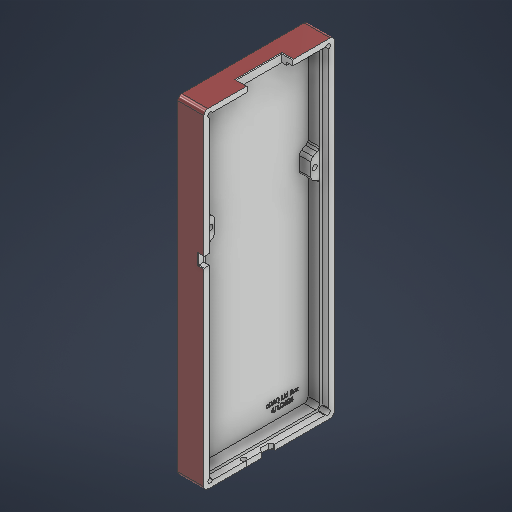
# Autodesk Inventor part: cDAQ_Lid_Box
Saved by Autodesk Inventor 2027 (Build 310192000, 192)
## iProperties
Created: 2026-05-08
Part Number: cDAQ_Lid_Box
Material: Generic
Document SubType Name: Modeling
Designer: giese
Density: 1 g/cm^3
Appearance: Default
Author: giese
Autodesk Inventor part; units mm, degrees
(part 1 of 2)
ref_plane "YZ Plane" through (0, 0, 0) normal (1, 0, 0) x (0, 1, 0)
ref_plane "XZ Plane" through (0, 0, 0) normal (0, 1, 0) x (-1, 0, 0)
ref_plane "XY Plane" through (0, 0, 0) normal (0, 0, 1) x (1, 0, 0)
sketch "Sketch1" plane through (0, 0, 0) normal (1, 0, 0) x (0, 1, 0)
  line L0 (50.7569, 48.4212) -> (-205.7831, 48.4212)
  line L1 (-205.7831, 48.4212) -> (-205.7831, -53.1788)
  line L2 (-205.7831, -53.1788) -> (50.7569, -53.1788)
  line L3 (50.7569, -53.1788) -> (50.7569, 48.4212)
  point P0 (0, 0)
  dimension "d0" = 101.6
  dimension "d1" = 256.54
  constraints: 8 end point, 2 parallel, 1 horizontal, 1 perpendicular
  measures "d0" distance of L2.end L0.start
  measures "d1" distance of L0.start L0.end
extrude "Extrusion1" add sketch "Sketch1" along normal blind 20.32
sketch "Sketch2" plane through (20.32, 0, 0) normal (1, 0, 0) x (0, 0, -1)
  line L0 (-42.0712, 44.4069) -> (46.8288, 44.4069)
  line L1 (46.8288, 44.4069) -> (46.8288, -199.4331)
  line L2 (46.8288, -199.4331) -> (-42.0712, -199.4331)
  line L3 (-42.0712, -199.4331) -> (-42.0712, 44.4069)
  line L4 (-48.4212, 50.7569) -> (-48.4212, -205.7831) projected
  line L5 (-48.4212, -205.7831) -> (53.1788, -205.7831) projected
  point P0 (0, 0)
  dimension "d4" = 88.9
  dimension "d5" = 243.84
  dimension "d6" = 6.35
  dimension "d7" = 6.35
  constraints: 8 end point, 2 parallel, 1 horizontal, 1 perpendicular
  measures "d4" distance of L0.start L0.end
  measures "d5" distance of L0.end L1.end
  measures "d6" distance between parallel lines of L4 L3
  measures "d7" distance between parallel lines of L5 L2
extrude "Extrusion2" cut sketch "Sketch2" against normal blind 13.97
sketch "Sketch3" plane through (0, 0, 0) normal (-1, 0, 0) x (0, 0, 1)
  circle A0 centre (-30.3188, 7.3229) radius 2
  line L0 (-53.1788, -205.7831) -> (-53.1788, 50.7569) projected
  line L1 (-53.1788, 50.7569) -> (48.4212, 50.7569) projected
  circle A1 centre (-11.82, 7.3229) radius 2
  circle A2 centre (6.6789, 7.3229) radius 2
  point P0 (0, 0)
  dimension "d10" = 22.86
  dimension "d11" = 43.434
  dimension "d12" = 43.434
  dimension "d13" = 18.4988
  dimension "d14" = 4
  dimension "d15" = 4
  dimension "d16" = 43.434
  dimension "d17" = 18.4988
  dimension "d18" = 36.9976
  dimension "d21" = 4
  constraints: 3 centre point
  measures "d10" distance from line of L0 A0.centre
  measures "d11" distance from line of L1 A0.centre
  measures "d12" distance from line of L1 A1.centre
  measures "d13" distance of A0.centre A1.centre
  measures "d14" diameter of A1
  measures "d15" diameter of A2
  measures "d16" distance from line of L1 A2.centre
  measures "d17" distance of A1.centre A2.centre
  measures "d18" distance of A0.centre A2.centre
  measures "d21" diameter of A0
extrude "Extrusion3" [suppressed]
sketch "Sketch6" plane through (0, 50.7569, 48.4212) normal (0, 1, 0) x (1, 0, 0)
  line L0 (20.32, 6.35) -> (20.32, 95.25) projected
  line L1 (11.684, 33.7719) -> (20.32, 33.7719)
  line L2 (20.32, 33.7719) -> (20.32, 69.342)
  line L3 (20.32, 69.342) -> (11.684, 69.342)
  line L4 (11.684, 69.342) -> (11.684, 33.7719)
  line L5 (0, 101.6) -> (20.32, 101.6) projected
  point P0 (0, 48.4212)
  point P1 (16.002, 69.342)
  point P2 (16.002, 33.7719)
  dimension "d30" = 8.636
  dimension "d31" = 35.5701
  dimension "d32" = 32.258
  constraints: 8 end point, 2 midpoint, 2 parallel, 1 horizontal, 1 perpendicular, 1 point on line
  measures "d30" distance between parallel lines of L0 L4
  measures "d31" distance of point (16.002, 69.342) point (16.002, 33.772)
  measures "d32" distance between parallel lines of L5 L3
extrude "Extrusion5" cut sketch "Sketch6" against normal blind 6.35
fillet "Fillet1" radius 3.175 4 edges at (10.16, 50.7569, -53.1788) (10.16, 50.7569, 48.4212) (10.16, -205.7831, 48.4212) (10.16, -205.7831, -53.1788)
sketch "Sketch7" plane through (20.32, 0, 0) normal (1, 0, 0) x (0, 0, -1)
  line L0 (-42.0712, -199.4331) -> (-42.0712, 44.4069) projected
  line L1 (-42.0712, 44.4069) -> (-42.3252, 44.4069)
  line L2 (-42.3252, 46.4643) -> (-44.1286, 46.4643)
  line L3 (-44.1286, 46.4643) -> (-44.1286, 51.0109)
  line L4 (-42.0712, -190.1621) -> (-42.0712, -199.4331)
  line L5 (46.8288, -199.4331) -> (-42.0712, -199.4331) projected
  line L6 (-40.4202, -201.4905) -> (-44.1286, -201.4905)
  line L7 (-44.1286, -201.4905) -> (-44.1286, -190.1621)
  line L8 (46.8288, 44.4069) -> (46.8288, -199.4331) projected
  line L9 (46.8288, -192.7021) -> (46.8288, -199.4331)
  line L10 (46.8288, -199.4331) -> (43.9078, -199.4331)
  line L11 (46.8288, -199.4331) -> (46.8288, -192.7021)
  line L12 (48.8862, -192.7021) -> (48.8862, -201.4905)
  line L13 (48.8862, -201.4905) -> (43.9078, -201.4905)
  line L14 (-42.0712, 44.4069) -> (46.8288, 44.4069) projected
  line L15 (42.0028, 44.4069) -> (46.8288, 44.4069)
  line L16 (48.8862, 48.4709) -> (48.8862, 46.4643)
  line L17 (48.8862, 46.4643) -> (42.0028, 46.4643)
  line L18 (-42.3252, 46.4643) -> (42.0028, 46.4643)
  line L19 (42.0028, 44.4069) -> (-42.3252, 44.4069)
  line L20 (48.8862, 48.4709) -> (48.8862, -192.7021)
  line L21 (44.2888, -195.2421) -> (44.2888, 44.4069)
  line L22 (43.9078, -199.4331) -> (-40.4202, -199.4331)
  line L23 (-40.4202, -201.4905) -> (43.9078, -201.4905)
  line L24 (-44.1286, -190.1621) -> (-44.1286, 51.0109)
  line L25 (-42.0712, 44.4069) -> (-42.0712, -190.1621)
  point P0 (0, 0)
  point P1 (-42.0712, 51.0109)
  point P2 (-44.2302, 48.9789)
  point P3 (46.8288, 48.4709)
  point P4 (48.8862, 46.4643)
  dimension "d34" = 2.0574
  dimension "d35" = 2.0574
  dimension "d38" = 2.0574
  dimension "d39" = 2.0574
  dimension "d42" = 2.0574
  dimension "d43" = 2.0574
  dimension "d46" = 2.0574
  dimension "d47" = 2.0574
  constraints: 44 end point, 9 point on line, 4 parallel, 4 perpendicular, 2 collinear, 2 horizontal, 2 vertical
  measures "d34" distance between parallel lines of L2 L1
  measures "d35" distance between parallel lines of L0 L3
  measures "d38" distance between parallel lines of L7 L0
  measures "d39" distance between parallel lines of L5 L6
  measures "d42" distance between parallel lines of L5 L13
  measures "d43" distance between parallel lines of L8 L12
  measures "d46" distance between parallel lines of L14 L17
  measures "d47" distance between parallel lines of L8 L16
extrude "Extrusion6" cut sketch "Sketch7" against normal blind 5 contours L0 L14 L8 L5 | L18 L17 L20 L12 L13 L23 L6 L7 L24 L2
fillet "Fillet2" radius 3.175 6 edges at (10.835, 44.4069, 42.0712) (10.835, 44.4069, -46.8288) (10.835, -199.4331, 42.0712) (17.82, -201.4905, 44.1286) (10.835, -199.4331, -46.8288) (17.82, -201.4905, -48.8862)
sketch "Sketch11" plane through (15.32, 0, 0) normal (1, 0, 0) x (0, 0, -1)
  circle A0 centre (48.0988, 45.6769) radius 1.9939
  line L0 (50.0038, 50.7569) -> (20.9208, 50.7569) projected
  line L1 (53.1788, -202.6081) -> (53.1788, 47.5819) projected
  arc A1 (46.9238, 45.7719) -> (43.7488, 48.9469) centre (43.7488, 45.7719) ccw projected
  circle A2 centre (-43.3412, 45.6769) radius 1.9939
  line L2 (-48.4212, 47.5819) -> (-48.4212, -202.6081) projected
  line L3 (-14.6493, 50.7569) -> (-45.2462, 50.7569) projected
  circle A3 centre (48.0988, -200.7031) radius 1.9939
  line L4 (-45.2462, -205.7831) -> (50.0038, -205.7831) projected
  circle A4 centre (-43.3412, -200.7031) radius 1.9939
  circle A5 centre (43.0188, -35.6031) radius 1.9939
  circle A6 centre (-38.2612, -35.6031) radius 1.9939
  point P0 (0, 0)
  point P1 (45.9939, 48.017)
  point P2 (48.5528, -43.2993)
  point P3 (45.3778, -46.4743)
  point P4 (-30.4007, -42.8803)
  point P5 (-33.5757, -46.0553)
  dimension "d58" = 3.9878
  dimension "d59" = 5.08
  dimension "d60" = 5.08
  dimension "d61" = 3.9878
  dimension "d62" = 3.9878
  dimension "d63" = 5.08
  dimension "d64" = 5.08
  dimension "d65" = 3.9878
  dimension "d66" = 5.08
  dimension "d67" = 5.08
  dimension "d76" = 5.08
  dimension "d77" = 5.08
  dimension "d114" = 3.9878
  dimension "d115" = 86.36
  dimension "d116" = 10.16
  dimension "d117" = 3.9878
  dimension "d118" = 86.36
  dimension "d119" = 10.16
  constraints: 6 centre point, 1 point on circle
  measures "d58" diameter of A0
  measures "d59" distance from line of L2 A2.centre
  measures "d60" distance from line of L3 A2.centre
  measures "d61" diameter of A2
  measures "d62" diameter of A3
  measures "d63" distance from line of L1 A3.centre
  measures "d64" distance from line of L4 A3.centre
  measures "d65" diameter of A4
  measures "d66" distance from line of L2 A4.centre
  measures "d67" distance from line of L4 A4.centre
  measures "d76" distance from line of L1 A0.centre
  measures "d77" distance from line of L0 A0.centre
  measures "d114" diameter of A5
  measures "d115" distance from line of A5.centre L0
  measures "d116" distance from line of L1 A5.centre
  measures "d117" diameter of A6
  measures "d118" distance from line of A6.centre L3
  measures "d119" distance from line of L2 A6.centre
extrude "Extrusion8" cut sketch "Sketch11" along normal blind 5.08 and the other way blind 17.78
sketch "Sketch13" plane through (6.35, 0, 0) normal (1, 0, 0) x (0, 0, -1)
  line L0 (14.1785, -185.2739) -> (39.2344, -185.2739) construction
  line L1 (39.2344, -185.2739) -> (39.2344, -194.1382) construction
  line L2 (39.2344, -194.1382) -> (14.1785, -194.1382) construction
  line L3 (14.1785, -194.1382) -> (14.1785, -185.2739) construction
  spline S0 degree 2 poles (15.3666, -188.5097) (15.1295, -188.5097) (14.7367, -188.3639) (14.5959, -188.2157) knots 0 0 0 1 2 2 2
  spline S1 degree 2 poles (14.5959, -188.2157) (14.4552, -188.07) (14.2995, -187.6205) (14.2995, -187.3191) knots 0 0 0 1 2 2 2
  spline S2 degree 2 poles (14.2995, -187.3191) (14.2995, -187.0178) (14.4601, -186.5781) (14.5959, -186.4299) knots 0 0 0 1 2 2 2
  spline S3 degree 2 poles (14.5959, -186.4299) (14.7318, -186.2792) (15.1344, -186.1187) (15.3666, -186.1187) knots 0 0 0 1 2 2 2
  spline S4 degree 2 poles (15.3666, -186.1187) (15.5543, -186.1187) (15.9051, -186.2249) (16.0409, -186.2941) knots 0 0 0 1 2 2 2
  line L4 (16.0409, -186.2941) -> (16.0409, -186.7263)
  line L5 (16.0409, -186.7263) -> (16.0187, -186.7263)
  spline S5 degree 2 poles (16.0187, -186.7263) (15.9767, -186.6917) (15.8482, -186.6028) (15.7569, -186.5559) knots 0 0 0 1 2 2 2
  spline S6 degree 2 poles (15.7569, -186.5559) (15.6753, -186.5164) (15.458, -186.4546) (15.3592, -186.4546) knots 0 0 0 1 2 2 2
  spline S7 degree 2 poles (15.3592, -186.4546) (15.0603, -186.4546) (14.6972, -186.9066) (14.6972, -187.3191) knots 0 0 0 1 2 2 2
  spline S8 degree 2 poles (14.6972, -187.3191) (14.6972, -187.7217) (15.048, -188.1737) (15.3592, -188.1737) knots 0 0 0 1 2 2 2
  spline S9 degree 2 poles (15.3592, -188.1737) (15.5469, -188.1737) (15.8878, -188.0181) (16.0187, -187.8971) knots 0 0 0 1 2 2 2
  line L6 (16.0187, -187.8971) -> (16.0409, -187.8971)
  line L7 (16.0409, -187.8971) -> (16.0409, -188.3293)
  spline S10 degree 2 poles (16.0409, -188.3293) (15.9841, -188.3565) (15.8112, -188.4331) (15.742, -188.4504) knots 0 0 0 1 2 2 2
  spline S11 degree 2 poles (15.742, -188.4504) (15.6432, -188.48) (15.4876, -188.5097) (15.3666, -188.5097) knots 0 0 0 1 2 2 2
  spline S12 degree 2 poles (18.8246, -186.9363) (18.8246, -187.3537) (18.4862, -188.0255) (18.2022, -188.2133) knots 0 0 0 1 2 2 2
  spline S13 degree 2 poles (18.2022, -188.2133) (17.97, -188.359) (17.4933, -188.4578) (17.1228, -188.4578) knots 0 0 0 1 2 2 2
  line L8 (17.1228, -188.4578) -> (16.4213, -188.4578)
  line L9 (16.4213, -188.4578) -> (16.4213, -185.4098)
  line L10 (16.4213, -185.4098) -> (17.1154, -185.4098)
  spline S14 degree 2 poles (17.1154, -185.4098) (17.5451, -185.4098) (18.0342, -185.5382) (18.2071, -185.6519) knots 0 0 0 1 2 2 2
  spline S15 degree 2 poles (18.2071, -185.6519) (18.501, -185.847) (18.8246, -186.4917) (18.8246, -186.9363) knots 0 0 0 1 2 2 2
  spline S16 degree 2 poles (18.4022, -186.9313) (18.4022, -186.5806) (18.1701, -186.0841) (17.9404, -185.9433) knots 0 0 0 1 2 2 2
  spline S17 degree 2 poles (17.9404, -185.9433) (17.7773, -185.847) (17.4093, -185.7605) (17.1351, -185.7605) knots 0 0 0 1 2 2 2
  line L11 (17.1351, -185.7605) -> (16.8264, -185.7605)
  line L12 (16.8264, -185.7605) -> (16.8264, -188.107)
  line L13 (16.8264, -188.107) -> (17.1351, -188.107)
  spline S18 degree 2 poles (17.1351, -188.107) (17.4044, -188.107) (17.8119, -188.0206) (17.9774, -187.9045) knots 0 0 0 1 2 2 2
  spline S19 degree 2 poles (17.9774, -187.9045) (18.1898, -187.7612) (18.4022, -187.287) (18.4022, -186.9313) knots 0 0 0 1 2 2 2
  line L14 (18.9358, -188.4578) -> (19.9633, -185.4098)
  line L15 (19.9633, -185.4098) -> (20.4622, -185.4098)
  line L16 (20.4622, -185.4098) -> (21.4898, -188.4578)
  line L17 (21.4898, -188.4578) -> (21.0625, -188.4578)
  line L18 (21.0625, -188.4578) -> (20.7858, -187.6056)
  line L19 (20.7858, -187.6056) -> (19.6224, -187.6056)
  line L20 (19.6224, -187.6056) -> (19.3458, -188.4578)
  line L21 (19.3458, -188.4578) -> (18.9358, -188.4578)
  line L22 (20.6747, -187.2598) -> (20.2029, -185.8248)
  line L23 (20.2029, -185.8248) -> (19.7336, -187.2598)
  line L24 (19.7336, -187.2598) -> (20.6747, -187.2598)
  spline S20 degree 2 poles (24.3105, -189.2037) (24.1994, -189.2309) (23.9573, -189.2605) (23.8363, -189.2605) knots 0 0 0 1 2 2 2
  spline S21 degree 2 poles (23.8363, -189.2605) (23.4929, -189.2605) (23.0656, -188.8777) (23.0459, -188.522) knots 0 0 0 1 2 2 2
  spline S22 degree 2 poles (23.0459, -188.522) (23.0187, -188.522) (22.9718, -188.522) (22.952, -188.522) knots 0 0 0 1 2 2 2
  spline S23 degree 2 poles (22.952, -188.522) (22.6433, -188.522) (22.1468, -188.3121) (21.9689, -188.107) knots 0 0 0 1 2 2 2
  spline S24 degree 2 poles (21.9689, -188.107) (21.7936, -187.9045) (21.6059, -187.3117) (21.6059, -186.9363) knots 0 0 0 1 2 2 2
  spline S25 degree 2 poles (21.6059, -186.9363) (21.6059, -186.5509) (21.796, -185.968) (21.9714, -185.7605) knots 0 0 0 1 2 2 2
  spline S26 degree 2 poles (21.9714, -185.7605) (22.1493, -185.5555) (22.6457, -185.3456) (22.952, -185.3456) knots 0 0 0 1 2 2 2
  spline S27 degree 2 poles (22.952, -185.3456) (23.2632, -185.3456) (23.7622, -185.5629) (23.9351, -185.7605) knots 0 0 0 1 2 2 2
  spline S28 degree 2 poles (23.9351, -185.7605) (24.108, -185.9606) (24.3006, -186.5559) (24.3006, -186.9363) knots 0 0 0 1 2 2 2
  spline S29 degree 2 poles (24.3006, -186.9363) (24.3006, -187.5291) (23.8387, -188.2997) (23.4361, -188.4356) knots 0 0 0 1 2 2 2
  spline S30 degree 2 poles (23.4361, -188.4356) (23.446, -188.5492) (23.5053, -188.732) (23.5522, -188.7838) knots 0 0 0 1 2 2 2
  spline S31 degree 2 poles (23.5522, -188.7838) (23.609, -188.8481) (23.7646, -188.9073) (23.903, -188.9073) knots 0 0 0 1 2 2 2
  spline S32 degree 2 poles (23.903, -188.9073) (23.9845, -188.9073) (24.2068, -188.8555) (24.2562, -188.8357) knots 0 0 0 1 2 2 2
  line L25 (24.2562, -188.8357) -> (24.3105, -188.8357)
  line L26 (24.3105, -188.8357) -> (24.3105, -189.2037)
  spline S33 degree 2 poles (23.8783, -186.9363) (23.8783, -186.6324) (23.7474, -186.1656) (23.6288, -186.0125) knots 0 0 0 1 2 2 2
  spline S34 degree 2 poles (23.6288, -186.0125) (23.5078, -185.8544) (23.1669, -185.6963) (22.9545, -185.6963) knots 0 0 0 1 2 2 2
  spline S35 degree 2 poles (22.9545, -185.6963) (22.7347, -185.6963) (22.4037, -185.8495) (22.2777, -186.0125) knots 0 0 0 1 2 2 2
  spline S36 degree 2 poles (22.2777, -186.0125) (22.1567, -186.1681) (22.0282, -186.6399) (22.0282, -186.9363) knots 0 0 0 1 2 2 2
  spline S37 degree 2 poles (22.0282, -186.9363) (22.0282, -187.5365) (22.5321, -188.1762) (22.9545, -188.1762) knots 0 0 0 1 2 2 2
  spline S38 degree 2 poles (22.9545, -188.1762) (23.3769, -188.1762) (23.8783, -187.5365) (23.8783, -186.9363) knots 0 0 0 1 2 2 2
  line L27 (27.8204, -188.4578) -> (26.0544, -188.4578)
  line L28 (26.0544, -188.4578) -> (26.0544, -185.4098)
  line L29 (26.0544, -185.4098) -> (26.4594, -185.4098)
  line L30 (26.4594, -185.4098) -> (26.4594, -188.0972)
  line L31 (26.4594, -188.0972) -> (27.8204, -188.0972)
  line L32 (27.8204, -188.0972) -> (27.8204, -188.4578)
  line L33 (28.5021, -188.4578) -> (28.1168, -188.4578)
  line L34 (28.1168, -188.4578) -> (28.1168, -186.1706)
  line L35 (28.1168, -186.1706) -> (28.5021, -186.1706)
  line L36 (28.5021, -186.1706) -> (28.5021, -188.4578)
  line L37 (28.5293, -185.7902) -> (28.0921, -185.7902)
  line L38 (28.0921, -185.7902) -> (28.0921, -185.39)
  line L39 (28.0921, -185.39) -> (28.5293, -185.39)
  line L40 (28.5293, -185.39) -> (28.5293, -185.7902)
  line L41 (30.8264, -188.4578) -> (30.4411, -188.4578)
  line L42 (30.4411, -188.4578) -> (30.4411, -188.2256)
  spline S39 degree 2 poles (30.4411, -188.2256) (30.3522, -188.2997) (30.2213, -188.3985) (30.1324, -188.4405) knots 0 0 0 1 2 2 2
  spline S40 degree 2 poles (30.1324, -188.4405) (30.0508, -188.48) (29.8755, -188.522) (29.7594, -188.522) knots 0 0 0 1 2 2 2
  spline S41 degree 2 poles (29.7594, -188.522) (29.5717, -188.522) (29.2555, -188.3664) (29.1443, -188.2157) knots 0 0 0 1 2 2 2
  spline S42 degree 2 poles (29.1443, -188.2157) (29.0332, -188.0651) (28.9097, -187.6205) (28.9097, -187.3315) knots 0 0 0 1 2 2 2
  spline S43 degree 2 poles (28.9097, -187.3315) (28.9097, -187.0301) (29.0653, -186.5905) (29.2012, -186.425) knots 0 0 0 1 2 2 2
  spline S44 degree 2 poles (29.2012, -186.425) (29.3271, -186.2768) (29.6803, -186.1063) (29.8755, -186.1063) knots 0 0 0 1 2 2 2
  spline S45 degree 2 poles (29.8755, -186.1063) (30.0459, -186.1063) (30.3003, -186.1829) (30.4411, -186.2619) knots 0 0 0 1 2 2 2
  line L43 (30.4411, -186.2619) -> (30.4411, -185.2739)
  line L44 (30.4411, -185.2739) -> (30.8264, -185.2739)
  line L45 (30.8264, -185.2739) -> (30.8264, -188.4578)
  line L46 (30.4411, -187.902) -> (30.4411, -186.5806)
  spline S46 degree 2 poles (30.4411, -186.5806) (30.2978, -186.5114) (30.0706, -186.4595) (29.9397, -186.4595) knots 0 0 0 1 2 2 2
  spline S47 degree 2 poles (29.9397, -186.4595) (29.6433, -186.4595) (29.3074, -186.9041) (29.3074, -187.3241) knots 0 0 0 1 2 2 2
  spline S48 degree 2 poles (29.3074, -187.3241) (29.3074, -187.7291) (29.5642, -188.1564) (29.8483, -188.1564) knots 0 0 0 1 2 2 2
  spline S49 degree 2 poles (29.8483, -188.1564) (29.999, -188.1564) (30.3053, -188.0181) (30.4411, -187.902) knots 0 0 0 1 2 2 2
  spline S50 degree 2 poles (34.7908, -187.5217) (34.7908, -187.7489) (34.6179, -188.0972) (34.4746, -188.2108) knots 0 0 0 1 2 2 2
  spline S51 degree 2 poles (34.4746, -188.2108) (34.3017, -188.3442) (33.909, -188.4578) (33.5978, -188.4578) knots 0 0 0 1 2 2 2
  line L47 (33.5978, -188.4578) -> (32.7234, -188.4578)
  line L48 (32.7234, -188.4578) -> (32.7234, -185.4098)
  line L49 (32.7234, -185.4098) -> (33.5311, -185.4098)
  spline S52 degree 2 poles (33.5311, -185.4098) (33.8571, -185.4098) (34.1832, -185.4518) (34.3314, -185.5333) knots 0 0 0 1 2 2 2
  spline S53 degree 2 poles (34.3314, -185.5333) (34.4969, -185.6197) (34.6475, -185.9038) (34.6475, -186.0965) knots 0 0 0 1 2 2 2
  spline S54 degree 2 poles (34.6475, -186.0965) (34.6475, -186.3113) (34.4203, -186.6522) (34.2202, -186.7485) knots 0 0 0 1 2 2 2
  line L50 (34.2202, -186.7485) -> (34.2202, -186.7634)
  spline S55 degree 2 poles (34.2202, -186.7634) (34.4919, -186.8375) (34.7908, -187.2302) (34.7908, -187.5217) knots 0 0 0 1 2 2 2
  spline S56 degree 2 poles (34.3684, -187.5389) (34.3684, -187.366) (34.2696, -187.1437) (34.1214, -187.0647) knots 0 0 0 1 2 2 2
  spline S57 degree 2 poles (34.1214, -187.0647) (34.0251, -187.0153) (33.7979, -186.9857) (33.5879, -186.9857) knots 0 0 0 1 2 2 2
  line L51 (33.5879, -186.9857) -> (33.1285, -186.9857)
  line L52 (33.1285, -186.9857) -> (33.1285, -188.112)
  line L53 (33.1285, -188.112) -> (33.457, -188.112)
  spline S58 degree 2 poles (33.457, -188.112) (33.7238, -188.112) (34.03, -188.0626) (34.1486, -187.9835) knots 0 0 0 1 2 2 2
  spline S59 degree 2 poles (34.1486, -187.9835) (34.2622, -187.902) (34.3684, -187.6995) (34.3684, -187.5389) knots 0 0 0 1 2 2 2
  spline S60 degree 2 poles (34.2252, -186.1533) (34.2252, -186.0446) (34.1511, -185.8816) (34.0696, -185.8346) knots 0 0 0 1 2 2 2
  spline S61 degree 2 poles (34.0696, -185.8346) (33.9708, -185.7803) (33.7312, -185.7556) (33.5163, -185.7556) knots 0 0 0 1 2 2 2
  line L54 (33.5163, -185.7556) -> (33.1285, -185.7556)
  line L55 (33.1285, -185.7556) -> (33.1285, -186.6473)
  line L56 (33.1285, -186.6473) -> (33.5879, -186.6473)
  spline S62 degree 2 poles (33.5879, -186.6473) (33.7781, -186.6473) (33.9584, -186.6077) (34.0547, -186.546) knots 0 0 0 1 2 2 2
  spline S63 degree 2 poles (34.0547, -186.546) (34.1486, -186.4867) (34.2252, -186.2965) (34.2252, -186.1533) knots 0 0 0 1 2 2 2
  spline S64 degree 2 poles (37.0435, -187.3142) (37.0435, -187.8922) (36.4877, -188.522) (36.0233, -188.522) knots 0 0 0 1 2 2 2
  spline S65 degree 2 poles (36.0233, -188.522) (35.5466, -188.522) (35.0008, -187.8724) (35.0008, -187.3142) knots 0 0 0 1 2 2 2
  spline S66 degree 2 poles (35.0008, -187.3142) (35.0008, -186.7411) (35.5639, -186.1063) (36.0233, -186.1063) knots 0 0 0 1 2 2 2
  spline S67 degree 2 poles (36.0233, -186.1063) (36.4877, -186.1063) (37.0435, -186.7387) (37.0435, -187.3142) knots 0 0 0 1 2 2 2
  spline S68 degree 2 poles (36.6458, -187.3142) (36.6458, -186.8696) (36.3222, -186.4373) (36.0233, -186.4373) knots 0 0 0 1 2 2 2
  spline S69 degree 2 poles (36.0233, -186.4373) (35.7245, -186.4373) (35.3984, -186.8696) (35.3984, -187.3142) knots 0 0 0 1 2 2 2
  spline S70 degree 2 poles (35.3984, -187.3142) (35.3984, -187.7464) (35.7245, -188.191) (36.0233, -188.191) knots 0 0 0 1 2 2 2
  spline S71 degree 2 poles (36.0233, -188.191) (36.3197, -188.191) (36.6458, -187.7538) (36.6458, -187.3142) knots 0 0 0 1 2 2 2
  line L57 (39.2146, -188.4578) -> (38.7428, -188.4578)
  line L58 (38.7428, -188.4578) -> (38.1871, -187.5982)
  line L59 (38.1871, -187.5982) -> (37.6165, -188.4578)
  line L60 (37.6165, -188.4578) -> (37.1793, -188.4578)
  line L61 (37.1793, -188.4578) -> (37.9722, -187.3241)
  line L62 (37.9722, -187.3241) -> (37.1867, -186.1706)
  line L63 (37.1867, -186.1706) -> (37.6585, -186.1706)
  line L64 (37.6585, -186.1706) -> (38.2118, -187.0227)
  line L65 (38.2118, -187.0227) -> (38.7774, -186.1706)
  line L66 (38.7774, -186.1706) -> (39.2146, -186.1706)
  line L67 (39.2146, -186.1706) -> (38.4267, -187.2994)
  line L68 (38.4267, -187.2994) -> (39.2146, -188.4578)
  spline S72 degree 2 poles (20.3906, -192.4882) (20.3906, -192.7229) (20.235, -193.1206) (20.1041, -193.2539) knots 0 0 0 1 2 2 2
  spline S73 degree 2 poles (20.1041, -193.2539) (19.9682, -193.3947) (19.6274, -193.5405) (19.4224, -193.5405) knots 0 0 0 1 2 2 2
  spline S74 degree 2 poles (19.4224, -193.5405) (19.2173, -193.5405) (18.879, -193.4021) (18.7505, -193.2638) knots 0 0 0 1 2 2 2
  spline S75 degree 2 poles (18.7505, -193.2638) (18.5924, -193.0983) (18.4146, -192.5426) (18.4146, -192.1375) knots 0 0 0 1 2 2 2
  spline S76 degree 2 poles (18.4146, -192.1375) (18.4146, -191.7398) (18.5776, -191.1001) (18.748, -190.863) knots 0 0 0 1 2 2 2
  spline S77 degree 2 poles (18.748, -190.863) (18.9135, -190.6308) (19.4372, -190.3714) (19.7805, -190.3714) knots 0 0 0 1 2 2 2
  spline S78 degree 2 poles (19.7805, -190.3714) (19.8818, -190.3714) (20.0596, -190.3912) (20.1263, -190.4134) knots 0 0 0 1 2 2 2
  line L69 (20.1263, -190.4134) -> (20.1263, -190.8062)
  line L70 (20.1263, -190.8062) -> (20.109, -190.8062)
  spline S79 degree 2 poles (20.109, -190.8062) (20.0522, -190.7765) (19.8447, -190.7246) (19.7262, -190.7246) knots 0 0 0 1 2 2 2
  spline S80 degree 2 poles (19.7262, -190.7246) (19.3458, -190.7246) (18.879, -191.2384) (18.8345, -191.7423) knots 0 0 0 1 2 2 2
  spline S81 degree 2 poles (18.8345, -191.7423) (18.9802, -191.641) (19.2865, -191.5299) (19.4693, -191.5299) knots 0 0 0 1 2 2 2
  spline S82 degree 2 poles (19.4693, -191.5299) (19.6471, -191.5299) (19.9139, -191.6015) (20.0596, -191.7102) knots 0 0 0 1 2 2 2
  spline S83 degree 2 poles (20.0596, -191.7102) (20.2276, -191.8362) (20.3906, -192.2264) (20.3906, -192.4882) knots 0 0 0 1 2 2 2
  spline S84 degree 2 poles (19.9756, -192.5055) (19.9756, -192.3178) (19.8768, -192.0634) (19.7682, -191.9745) knots 0 0 0 1 2 2 2
  spline S85 degree 2 poles (19.7682, -191.9745) (19.6867, -191.9103) (19.4841, -191.8683) (19.3779, -191.8683) knots 0 0 0 1 2 2 2
  spline S86 degree 2 poles (19.3779, -191.8683) (19.2346, -191.8683) (18.9654, -191.9547) (18.8345, -192.0362) knots 0 0 0 1 2 2 2
  spline S87 degree 2 poles (18.8345, -192.0362) (18.832, -192.0807) (18.8271, -192.1647) (18.8271, -192.2289) knots 0 0 0 1 2 2 2
  spline S88 degree 2 poles (18.8271, -192.2289) (18.8271, -192.545) (18.9506, -192.9328) (19.0444, -193.0341) knots 0 0 0 1 2 2 2
  spline S89 degree 2 poles (19.0444, -193.0341) (19.1309, -193.1304) (19.3186, -193.207) (19.4248, -193.207) knots 0 0 0 1 2 2 2
  spline S90 degree 2 poles (19.4248, -193.207) (19.6718, -193.207) (19.9756, -192.8563) (19.9756, -192.5055) knots 0 0 0 1 2 2 2
  line L71 (22.0183, -190.2924) -> (20.8253, -194.1382)
  line L72 (20.8253, -194.1382) -> (20.4795, -194.1382)
  line L73 (20.4795, -194.1382) -> (21.6676, -190.2924)
  line L74 (21.6676, -190.2924) -> (22.0183, -190.2924)
  line L75 (24.0808, -193.4762) -> (22.5939, -193.4762)
  line L76 (22.5939, -193.4762) -> (22.5939, -193.165)
  line L77 (22.5939, -193.165) -> (23.1471, -193.165)
  line L78 (23.1471, -193.165) -> (23.1471, -191.1223)
  line L79 (23.1471, -191.1223) -> (22.5939, -191.1223)
  line L80 (22.5939, -191.1223) -> (22.5939, -190.8432)
  spline S91 degree 2 poles (22.5939, -190.8432) (22.9076, -190.8432) (23.204, -190.6654) (23.2237, -190.4184) knots 0 0 0 1 2 2 2
  line L81 (23.2237, -190.4184) -> (23.5399, -190.4184)
  line L82 (23.5399, -190.4184) -> (23.5399, -193.165)
  line L83 (23.5399, -193.165) -> (24.0808, -193.165)
  line L84 (24.0808, -193.165) -> (24.0808, -193.4762)
  line L85 (25.9086, -190.2924) -> (24.7156, -194.1382)
  line L86 (24.7156, -194.1382) -> (24.3698, -194.1382)
  line L87 (24.3698, -194.1382) -> (25.5579, -190.2924)
  line L88 (25.5579, -190.2924) -> (25.9086, -190.2924)
  line L89 (28.1242, -193.4762) -> (26.2445, -193.4762)
  line L90 (26.2445, -193.4762) -> (26.2445, -193.044)
  spline S92 degree 2 poles (26.2445, -193.044) (26.4471, -192.8538) (26.8077, -192.5006) (26.9806, -192.3104) knots 0 0 0 1 2 2 2
  spline S93 degree 2 poles (26.9806, -192.3104) (27.3289, -191.9275) (27.5833, -191.4681) (27.5833, -191.2236) knots 0 0 0 1 2 2 2
  spline S94 degree 2 poles (27.5833, -191.2236) (27.5833, -191.0951) (27.5043, -190.9025) (27.4326, -190.8407) knots 0 0 0 1 2 2 2
  spline S95 degree 2 poles (27.4326, -190.8407) (27.361, -190.779) (27.1733, -190.7172) (27.0597, -190.7172) knots 0 0 0 1 2 2 2
  spline S96 degree 2 poles (27.0597, -190.7172) (26.951, -190.7172) (26.7287, -190.7716) (26.6274, -190.8136) knots 0 0 0 1 2 2 2
  spline S97 degree 2 poles (26.6274, -190.8136) (26.5409, -190.8481) (26.3804, -190.9469) (26.331, -190.9815) knots 0 0 0 1 2 2 2
  line L91 (26.331, -190.9815) -> (26.3088, -190.9815)
  line L92 (26.3088, -190.9815) -> (26.3088, -190.5468)
  spline S98 degree 2 poles (26.3088, -190.5468) (26.4347, -190.4851) (26.8867, -190.364) (27.0893, -190.364) knots 0 0 0 1 2 2 2
  spline S99 degree 2 poles (27.0893, -190.364) (27.5166, -190.364) (27.9983, -190.816) (27.9983, -191.2014) knots 0 0 0 1 2 2 2
  spline S100 degree 2 poles (27.9983, -191.2014) (27.9983, -191.3817) (27.9143, -191.683) (27.8402, -191.8114) knots 0 0 0 1 2 2 2
  spline S101 degree 2 poles (27.8402, -191.8114) (27.7661, -191.9448) (27.5512, -192.2067) (27.4326, -192.3326) knots 0 0 0 1 2 2 2
  spline S102 degree 2 poles (27.4326, -192.3326) (27.24, -192.5426) (26.7682, -192.9921) (26.6274, -193.123) knots 0 0 0 1 2 2 2
  line L93 (26.6274, -193.123) -> (28.1242, -193.123)
  line L94 (28.1242, -193.123) -> (28.1242, -193.4762)
  spline S103 degree 2 poles (30.4288, -191.9522) (30.4288, -192.7723) (29.952, -193.5405) (29.4556, -193.5405) knots 0 0 0 1 2 2 2
  spline S104 degree 2 poles (29.4556, -193.5405) (28.9517, -193.5405) (28.4799, -192.7575) (28.4799, -191.9547) knots 0 0 0 1 2 2 2
  spline S105 degree 2 poles (28.4799, -191.9547) (28.4799, -191.1297) (28.9566, -190.3665) (29.4556, -190.3665) knots 0 0 0 1 2 2 2
  spline S106 degree 2 poles (29.4556, -190.3665) (29.957, -190.3665) (30.4288, -191.1569) (30.4288, -191.9522) knots 0 0 0 1 2 2 2
  spline S107 degree 2 poles (29.9051, -192.881) (29.9644, -192.7303) (30.0138, -192.2659) (30.0138, -191.9522) knots 0 0 0 1 2 2 2
  spline S108 degree 2 poles (30.0138, -191.9522) (30.0138, -191.6385) (29.9644, -191.1767) (29.9026, -191.021) knots 0 0 0 1 2 2 2
  spline S109 degree 2 poles (29.9026, -191.021) (29.8409, -190.8654) (29.626, -190.7049) (29.4556, -190.7049) knots 0 0 0 1 2 2 2
  spline S110 degree 2 poles (29.4556, -190.7049) (29.2851, -190.7049) (29.0653, -190.8654) (29.0011, -191.026) knots 0 0 0 1 2 2 2
  spline S111 degree 2 poles (29.0011, -191.026) (28.9393, -191.1816) (28.8949, -191.6558) (28.8949, -191.9547) knots 0 0 0 1 2 2 2
  spline S112 degree 2 poles (28.8949, -191.9547) (28.8949, -192.2758) (28.9344, -192.7056) (28.9986, -192.8736) knots 0 0 0 1 2 2 2
  spline S113 degree 2 poles (28.9986, -192.8736) (29.0579, -193.0316) (29.2777, -193.2021) (29.4556, -193.2021) knots 0 0 0 1 2 2 2
  spline S114 degree 2 poles (29.4556, -193.2021) (29.6235, -193.2021) (29.8434, -193.0415) (29.9051, -192.881) knots 0 0 0 1 2 2 2
  line L95 (32.6987, -193.4762) -> (30.819, -193.4762)
  line L96 (30.819, -193.4762) -> (30.819, -193.044)
  spline S115 degree 2 poles (30.819, -193.044) (31.0216, -192.8538) (31.3822, -192.5006) (31.5551, -192.3104) knots 0 0 0 1 2 2 2
  spline S116 degree 2 poles (31.5551, -192.3104) (31.9034, -191.9275) (32.1578, -191.4681) (32.1578, -191.2236) knots 0 0 0 1 2 2 2
  spline S117 degree 2 poles (32.1578, -191.2236) (32.1578, -191.0951) (32.0787, -190.9025) (32.0071, -190.8407) knots 0 0 0 1 2 2 2
  spline S118 degree 2 poles (32.0071, -190.8407) (31.9355, -190.779) (31.7477, -190.7172) (31.6341, -190.7172) knots 0 0 0 1 2 2 2
  spline S119 degree 2 poles (31.6341, -190.7172) (31.5254, -190.7172) (31.3031, -190.7716) (31.2019, -190.8136) knots 0 0 0 1 2 2 2
  spline S120 degree 2 poles (31.2019, -190.8136) (31.1154, -190.8481) (30.9549, -190.9469) (30.9055, -190.9815) knots 0 0 0 1 2 2 2
  line L97 (30.9055, -190.9815) -> (30.8832, -190.9815)
  line L98 (30.8832, -190.9815) -> (30.8832, -190.5468)
  spline S121 degree 2 poles (30.8832, -190.5468) (31.0092, -190.4851) (31.4612, -190.364) (31.6638, -190.364) knots 0 0 0 1 2 2 2
  spline S122 degree 2 poles (31.6638, -190.364) (32.0911, -190.364) (32.5727, -190.816) (32.5727, -191.2014) knots 0 0 0 1 2 2 2
  spline S123 degree 2 poles (32.5727, -191.2014) (32.5727, -191.3817) (32.4887, -191.683) (32.4146, -191.8114) knots 0 0 0 1 2 2 2
  spline S124 degree 2 poles (32.4146, -191.8114) (32.3405, -191.9448) (32.1257, -192.2067) (32.0071, -192.3326) knots 0 0 0 1 2 2 2
  spline S125 degree 2 poles (32.0071, -192.3326) (31.8144, -192.5426) (31.3427, -192.9921) (31.2019, -193.123) knots 0 0 0 1 2 2 2
  line L99 (31.2019, -193.123) -> (32.6987, -193.123)
  line L100 (32.6987, -193.123) -> (32.6987, -193.4762)
  spline S126 degree 2 poles (35.0329, -192.4882) (35.0329, -192.7229) (34.8773, -193.1206) (34.7463, -193.2539) knots 0 0 0 1 2 2 2
  spline S127 degree 2 poles (34.7463, -193.2539) (34.6105, -193.3947) (34.2696, -193.5405) (34.0646, -193.5405) knots 0 0 0 1 2 2 2
  spline S128 degree 2 poles (34.0646, -193.5405) (33.8596, -193.5405) (33.5212, -193.4021) (33.3928, -193.2638) knots 0 0 0 1 2 2 2
  spline S129 degree 2 poles (33.3928, -193.2638) (33.2347, -193.0983) (33.0569, -192.5426) (33.0569, -192.1375) knots 0 0 0 1 2 2 2
  spline S130 degree 2 poles (33.0569, -192.1375) (33.0569, -191.7398) (33.2199, -191.1001) (33.3903, -190.863) knots 0 0 0 1 2 2 2
  spline S131 degree 2 poles (33.3903, -190.863) (33.5558, -190.6308) (34.0794, -190.3714) (34.4228, -190.3714) knots 0 0 0 1 2 2 2
  spline S132 degree 2 poles (34.4228, -190.3714) (34.524, -190.3714) (34.7019, -190.3912) (34.7686, -190.4134) knots 0 0 0 1 2 2 2
  line L101 (34.7686, -190.4134) -> (34.7686, -190.8062)
  line L102 (34.7686, -190.8062) -> (34.7513, -190.8062)
  spline S133 degree 2 poles (34.7513, -190.8062) (34.6945, -190.7765) (34.487, -190.7246) (34.3684, -190.7246) knots 0 0 0 1 2 2 2
  spline S134 degree 2 poles (34.3684, -190.7246) (33.988, -190.7246) (33.5212, -191.2384) (33.4768, -191.7423) knots 0 0 0 1 2 2 2
  spline S135 degree 2 poles (33.4768, -191.7423) (33.6225, -191.641) (33.9288, -191.5299) (34.1115, -191.5299) knots 0 0 0 1 2 2 2
  spline S136 degree 2 poles (34.1115, -191.5299) (34.2894, -191.5299) (34.5562, -191.6015) (34.7019, -191.7102) knots 0 0 0 1 2 2 2
  spline S137 degree 2 poles (34.7019, -191.7102) (34.8698, -191.8362) (35.0329, -192.2264) (35.0329, -192.4882) knots 0 0 0 1 2 2 2
  spline S138 degree 2 poles (34.6179, -192.5055) (34.6179, -192.3178) (34.5191, -192.0634) (34.4104, -191.9745) knots 0 0 0 1 2 2 2
  spline S139 degree 2 poles (34.4104, -191.9745) (34.3289, -191.9103) (34.1264, -191.8683) (34.0202, -191.8683) knots 0 0 0 1 2 2 2
  spline S140 degree 2 poles (34.0202, -191.8683) (33.8769, -191.8683) (33.6077, -191.9547) (33.4768, -192.0362) knots 0 0 0 1 2 2 2
  spline S141 degree 2 poles (33.4768, -192.0362) (33.4743, -192.0807) (33.4693, -192.1647) (33.4693, -192.2289) knots 0 0 0 1 2 2 2
  spline S142 degree 2 poles (33.4693, -192.2289) (33.4693, -192.545) (33.5928, -192.9328) (33.6867, -193.0341) knots 0 0 0 1 2 2 2
  spline S143 degree 2 poles (33.6867, -193.0341) (33.7732, -193.1304) (33.9609, -193.207) (34.0671, -193.207) knots 0 0 0 1 2 2 2
  spline S144 degree 2 poles (34.0671, -193.207) (34.3141, -193.207) (34.6179, -192.8563) (34.6179, -192.5055) knots 0 0 0 1 2 2 2
  point P0 (0, 0)
  constraints: 2 other
emboss "Emboss1" sketch "Sketch13" operation cut depth 2.54 direction (-1, 0, 0)
sketch "Sketch14" plane through (0, 0, 0) normal (-1, 0, 0) x (0, 0, 1)
  line L0 (-10.4499, -187.9273) -> (8.7669, -187.9273) construction
  line L1 (8.7669, -187.9273) -> (8.7669, -196.7101) construction
  line L2 (8.7669, -196.7101) -> (-10.4499, -196.7101) construction
  line L3 (-10.4499, -196.7101) -> (-10.4499, -187.9273) construction
  line L4 (-23.4175, -195.887) -> (-20.8486, -188.267)
  line L5 (-20.8486, -188.267) -> (-19.6013, -188.267)
  line L6 (-19.6013, -188.267) -> (-17.0325, -195.887)
  line L7 (-17.0325, -195.887) -> (-18.1008, -195.887)
  line L8 (-18.1008, -195.887) -> (-18.7924, -193.7566)
  line L9 (-18.7924, -193.7566) -> (-21.7008, -193.7566)
  line L10 (-21.7008, -193.7566) -> (-22.3924, -195.887)
  line L11 (-22.3924, -195.887) -> (-23.4175, -195.887)
  line L12 (-19.0702, -192.8921) -> (-20.2497, -189.3044)
  line L13 (-20.2497, -189.3044) -> (-21.4229, -192.8921)
  line L14 (-21.4229, -192.8921) -> (-19.0702, -192.8921)
  line L15 (-10.4128, -195.887) -> (-11.7281, -195.887)
  line L16 (-11.7281, -195.887) -> (-14.1364, -192.855)
  line L17 (-14.1364, -192.855) -> (-15.2973, -192.855)
  line L18 (-15.2973, -192.855) -> (-15.2973, -195.887)
  line L19 (-15.2973, -195.887) -> (-16.31, -195.887)
  line L20 (-16.31, -195.887) -> (-16.31, -188.267)
  line L21 (-16.31, -188.267) -> (-14.3463, -188.267)
  spline S0 degree 2 poles (-14.3463, -188.267) (-13.6918, -188.267) (-12.8087, -188.409) (-12.4074, -188.6683) knots 0 0 0 1 2 2 2
  spline S1 degree 2 poles (-12.4074, -188.6683) (-12.006, -188.9277) (-11.5429, -189.7366) (-11.5429, -190.3356) knots 0 0 0 1 2 2 2
  spline S2 degree 2 poles (-11.5429, -190.3356) (-11.5429, -191.1692) (-12.395, -192.2993) (-13.1237, -192.571) knots 0 0 0 1 2 2 2
  line L22 (-13.1237, -192.571) -> (-10.4128, -195.887)
  spline S3 degree 2 poles (-12.5988, -190.4159) (-12.5988, -190.0824) (-12.8334, -189.5699) (-13.0804, -189.4032) knots 0 0 0 1 2 2 2
  spline S4 degree 2 poles (-13.0804, -189.4032) (-13.2966, -189.2612) (-13.8708, -189.1438) (-14.2907, -189.1438) knots 0 0 0 1 2 2 2
  line L23 (-14.2907, -189.1438) -> (-15.2973, -189.1438)
  line L24 (-15.2973, -189.1438) -> (-15.2973, -192.009)
  line L25 (-15.2973, -192.009) -> (-14.4081, -192.009)
  spline S5 degree 2 poles (-14.4081, -192.009) (-13.9696, -192.009) (-13.2719, -191.8547) (-13.031, -191.6138) knots 0 0 0 1 2 2 2
  spline S6 degree 2 poles (-13.031, -191.6138) (-12.8087, -191.4039) (-12.5988, -190.8111) (-12.5988, -190.4159) knots 0 0 0 1 2 2 2
  line L26 (-8.0293, -195.887) -> (-8.0293, -189.1685)
  line L27 (-8.0293, -189.1685) -> (-10.5857, -189.1685)
  line L28 (-10.5857, -189.1685) -> (-10.5857, -188.267)
  line L29 (-10.5857, -188.267) -> (-4.4601, -188.267)
  line L30 (-4.4601, -188.267) -> (-4.4601, -189.1685)
  line L31 (-4.4601, -189.1685) -> (-7.0166, -189.1685)
  line L32 (-7.0166, -189.1685) -> (-7.0166, -195.887)
  line L33 (-7.0166, -195.887) -> (-8.0293, -195.887)
  spline S7 degree 2 poles (-1.564, -196.0228) (-2.3914, -196.0228) (-3.5524, -195.677) (-4.0649, -195.43) knots 0 0 0 1 2 2 2
  line L34 (-4.0649, -195.43) -> (-4.0649, -194.158)
  line L35 (-4.0649, -194.158) -> (-3.9908, -194.158)
  spline S8 degree 2 poles (-3.9908, -194.158) (-3.4906, -194.6273) (-2.2247, -195.146) (-1.6381, -195.146) knots 0 0 0 1 2 2 2
  spline S9 degree 2 poles (-1.6381, -195.146) (-0.7983, -195.146) (0.06, -194.4482) (0.06, -193.8739) knots 0 0 0 1 2 2 2
  spline S10 degree 2 poles (0.06, -193.8739) (0.06, -193.417) (-0.3907, -192.8489) (-0.8786, -192.7068) knots 0 0 0 1 2 2 2
  spline S11 degree 2 poles (-0.8786, -192.7068) (-1.2305, -192.608) (-1.8172, -192.4722) (-2.2556, -192.361) knots 0 0 0 1 2 2 2
  spline S12 degree 2 poles (-2.2556, -192.361) (-2.6508, -192.256) (-3.2745, -191.9411) (-3.5153, -191.6879) knots 0 0 0 1 2 2 2
  spline S13 degree 2 poles (-3.5153, -191.6879) (-3.75, -191.4348) (-4.0093, -190.7555) (-4.0093, -190.3109) knots 0 0 0 1 2 2 2
  spline S14 degree 2 poles (-4.0093, -190.3109) (-4.0093, -189.3847) (-2.5643, -188.1311) (-1.4467, -188.1311) knots 0 0 0 1 2 2 2
  spline S15 degree 2 poles (-1.4467, -188.1311) (-0.8045, -188.1311) (0.3317, -188.3843) (0.8196, -188.6251) knots 0 0 0 1 2 2 2
  line L36 (0.8196, -188.6251) -> (0.8196, -189.8354)
  line L37 (0.8196, -189.8354) -> (0.7455, -189.8354)
  spline S16 degree 2 poles (0.7455, -189.8354) (0.3811, -189.502) (-0.7551, -189.008) (-1.3787, -189.008) knots 0 0 0 1 2 2 2
  spline S17 degree 2 poles (-1.3787, -189.008) (-2.0827, -189.008) (-2.9534, -189.6687) (-2.9534, -190.2059) knots 0 0 0 1 2 2 2
  spline S18 degree 2 poles (-2.9534, -190.2059) (-2.9534, -190.6876) (-2.4408, -191.2619) (-1.9592, -191.3915) knots 0 0 0 1 2 2 2
  spline S19 degree 2 poles (-1.9592, -191.3915) (-1.6381, -191.478) (-0.7057, -191.7003) (-0.3969, -191.7929) knots 0 0 0 1 2 2 2
  spline S20 degree 2 poles (-0.3969, -191.7929) (0.3873, -192.0337) (1.116, -193.0032) (1.116, -193.7134) knots 0 0 0 1 2 2 2
  spline S21 degree 2 poles (1.116, -193.7134) (1.116, -194.1641) (0.7516, -195.0286) (0.4244, -195.3312) knots 0 0 0 1 2 2 2
  spline S22 degree 2 poles (0.4244, -195.3312) (0.06, -195.6647) (-0.8662, -196.0228) (-1.564, -196.0228) knots 0 0 0 1 2 2 2
  line L38 (4.7222, -193.0156) -> (1.8385, -193.0156)
  line L39 (1.8385, -193.0156) -> (1.8385, -192.0893)
  line L40 (1.8385, -192.0893) -> (4.7222, -192.0893)
  line L41 (4.7222, -192.0893) -> (4.7222, -193.0156)
  line L42 (10.3662, -195.887) -> (5.951, -195.887)
  line L43 (5.951, -195.887) -> (5.951, -188.267)
  line L44 (5.951, -188.267) -> (6.9637, -188.267)
  line L45 (6.9637, -188.267) -> (6.9637, -194.9854)
  line L46 (6.9637, -194.9854) -> (10.3662, -194.9854)
  line L47 (10.3662, -194.9854) -> (10.3662, -195.887)
  spline S23 degree 2 poles (14.275, -195.2818) (14.1577, -195.3683) (13.7625, -195.677) (13.5772, -195.7696) knots 0 0 0 1 2 2 2
  spline S24 degree 2 poles (13.5772, -195.7696) (13.324, -195.9055) (12.8486, -196.0475) (12.4163, -196.0475) knots 0 0 0 1 2 2 2
  spline S25 degree 2 poles (12.4163, -196.0475) (12.0643, -196.0475) (11.4283, -195.782) (11.1875, -195.5412) knots 0 0 0 1 2 2 2
  spline S26 degree 2 poles (11.1875, -195.5412) (10.959, -195.3065) (10.6811, -194.6149) (10.6811, -194.2321) knots 0 0 0 1 2 2 2
  spline S27 degree 2 poles (10.6811, -194.2321) (10.6811, -193.6393) (11.1813, -192.7995) (11.7247, -192.5586) knots 0 0 0 1 2 2 2
  spline S28 degree 2 poles (11.7247, -192.5586) (12.2063, -192.3363) (13.5155, -192.1696) (14.275, -192.1264) knots 0 0 0 1 2 2 2
  line L48 (14.275, -192.1264) -> (14.275, -191.9411)
  spline S29 degree 2 poles (14.275, -191.9411) (14.275, -191.6077) (14.0712, -191.1939) (13.886, -191.0766) knots 0 0 0 1 2 2 2
  spline S30 degree 2 poles (13.886, -191.0766) (13.7007, -190.9593) (13.1697, -190.8852) (12.8856, -190.8852) knots 0 0 0 1 2 2 2
  spline S31 degree 2 poles (12.8856, -190.8852) (12.5522, -190.8852) (11.6506, -191.0828) (11.1998, -191.2742) knots 0 0 0 1 2 2 2
  line L49 (11.1998, -191.2742) -> (11.1442, -191.2742)
  line L50 (11.1442, -191.2742) -> (11.1442, -190.2924)
  spline S32 degree 2 poles (11.1442, -190.2924) (11.4098, -190.2183) (12.404, -190.033) (12.8918, -190.033) knots 0 0 0 1 2 2 2
  spline S33 degree 2 poles (12.8918, -190.033) (13.4846, -190.033) (14.2935, -190.2183) (14.6146, -190.4591) knots 0 0 0 1 2 2 2
  spline S34 degree 2 poles (14.6146, -190.4591) (14.9295, -190.6938) (15.2383, -191.4409) (15.2383, -191.9782) knots 0 0 0 1 2 2 2
  line L51 (15.2383, -191.9782) -> (15.2383, -195.887)
  line L52 (15.2383, -195.887) -> (14.275, -195.887)
  line L53 (14.275, -195.887) -> (14.275, -195.2818)
  line L54 (14.275, -194.4791) -> (14.275, -192.8921)
  spline S35 degree 2 poles (14.275, -192.8921) (13.9292, -192.923) (12.8856, -193.0279) (12.5583, -193.1267) knots 0 0 0 1 2 2 2
  spline S36 degree 2 poles (12.5583, -193.1267) (12.1755, -193.2441) (11.6753, -193.7319) (11.6753, -194.1641) knots 0 0 0 1 2 2 2
  spline S37 degree 2 poles (11.6753, -194.1641) (11.6753, -194.6581) (12.231, -195.1583) (12.7621, -195.1583) knots 0 0 0 1 2 2 2
  spline S38 degree 2 poles (12.7621, -195.1583) (13.2129, -195.1583) (13.9539, -194.7693) (14.275, -194.4791) knots 0 0 0 1 2 2 2
  spline S39 degree 2 poles (21.3825, -192.9353) (21.3825, -194.337) (20.024, -196.0475) (18.9989, -196.0475) knots 0 0 0 1 2 2 2
  spline S40 degree 2 poles (18.9989, -196.0475) (18.5358, -196.0475) (17.875, -195.819) (17.5539, -195.6214) knots 0 0 0 1 2 2 2
  line L55 (17.5539, -195.6214) -> (17.4922, -195.887)
  line L56 (17.4922, -195.887) -> (16.5906, -195.887)
  line L57 (16.5906, -195.887) -> (16.5906, -187.9273)
  line L58 (16.5906, -187.9273) -> (17.5539, -187.9273)
  line L59 (17.5539, -187.9273) -> (17.5539, -190.7679)
  spline S41 degree 2 poles (17.5539, -190.7679) (17.9183, -190.4406) (18.7642, -190.0083) (19.3015, -190.0083) knots 0 0 0 1 2 2 2
  spline S42 degree 2 poles (19.3015, -190.0083) (20.271, -190.0083) (21.3825, -191.5583) (21.3825, -192.9353) knots 0 0 0 1 2 2 2
  spline S43 degree 2 poles (20.3883, -193.0094) (20.3883, -191.9843) (19.7646, -190.9222) (19.073, -190.9222) knots 0 0 0 1 2 2 2
  spline S44 degree 2 poles (19.073, -190.9222) (18.684, -190.9222) (17.8812, -191.2927) (17.5539, -191.5768) knots 0 0 0 1 2 2 2
  line L60 (17.5539, -191.5768) -> (17.5539, -194.8557)
  spline S45 degree 2 poles (17.5539, -194.8557) (17.9183, -195.0348) (18.4802, -195.183) (18.8136, -195.183) knots 0 0 0 1 2 2 2
  spline S46 degree 2 poles (18.8136, -195.183) (19.5485, -195.183) (20.3883, -194.1394) (20.3883, -193.0094) knots 0 0 0 1 2 2 2
  point P0 (0, 0)
  constraints: 2 other
emboss "Emboss2" sketch "Sketch14" operation cut depth 2.54 direction (1, 0, 0)
sketch "Sketch15" plane through (0, -202.6081, 48.4212) normal (0, 0, 1) x (1, 0, 0)
  line L0 (20.32, 0) -> (20.32, 250.19) projected
  line L1 (16.002, 147.1168) -> (20.32, 147.1168)
  line L2 (20.32, 147.1168) -> (20.32, 155.1178)
  line L3 (20.32, 155.1178) -> (16.002, 155.1178)
  line L4 (16.002, 155.1178) -> (16.002, 147.1168)
  line L5 (20.32, 253.365) -> (0, 253.365) projected
  point P0 (0, 202.6081)
  point P1 (18.161, 155.1178)
  dimension "d78" = 8.001
  dimension "d79" = 4.318
  dimension "d83" = 106.2482
  constraints: 8 end point, 2 parallel, 1 horizontal, 1 midpoint, 1 perpendicular, 1 point on line
  measures "d78" distance of L3.end L1.start
  measures "d79" distance between parallel lines of L0 L4
  measures "d83" distance between parallel lines of L5 L1
extrude "Extrusion9" cut sketch "Sketch15" against normal blind 6.35
sketch "Sketch18" plane through (0, -205.7831, -50.0038) normal (0, -1, 0) x (1, 0, 0)
  line L0 (20.32, 43.2816) -> (20.32, 53.2892)
  line L1 (20.32, 53.2892) -> (19.1008, 53.2892)
  line L2 (19.1008, 53.2892) -> (17.3482, 51.2892)
  line L3 (17.3482, 45.2816) -> (17.3482, 51.2892)
  line L4 (20.32, 98.425) -> (0, 98.425) projected
  line L5 (20.32, 95.25) -> (20.32, 0) projected
  line L6 (20.32, 43.2816) -> (19.1008, 43.2816)
  line L7 (19.1008, 43.2816) -> (17.3482, 45.2816)
  point P0 (19.7104, 53.2892)
  dimension "d91" = 1.2192
  dimension "d92" = 2
  dimension "d94" = 6.0076
  dimension "d95" = 10.0076
  dimension "d98" = 1.7526
  dimension "d99" = 0
  dimension "d165" = 45.1358
  constraints: 12 end point, 1 horizontal, 1 midpoint
  measures "d91" distance of L0.end L1.end
  measures "d92" vertical distance of L1.end L2.end
  measures "d94" distance of L3.start L2.end
  measures "d95" distance of L0.start L0.end
  measures "d98" distance from line of L1.end L3
  measures "d99" distance between parallel lines of L5 L0
  measures "d165" distance from line of L4 point (19.71, 53.289)
extrude "Extrusion10" cut sketch "Sketch18" against normal blind 6.35
sketch "Sketch19" plane through (0, 13.9785, -4.7779) normal (-1, 0, 0) x (0, 0, 1)
  arc A0 (-41.489, 32.4859) -> (-44.1083, 29.8666) centre (-43.3209, 31.6985) ccw projected
  circle A1 centre (-43.3209, 31.6985) radius 4.5085
  arc A2 (46.2873, 32.4859) -> (48.9065, 29.8666) centre (48.1191, 31.6985) ccw projected
  circle A3 centre (48.1191, 31.6985) radius 4.5085
  circle A4 centre (-43.3209, -214.6815) radius 1.9939 projected
  circle A5 centre (-43.3209, -214.6815) radius 4.5085
  arc A6 (46.2683, -215.4232) -> (48.8608, -212.8307) centre (48.1191, -214.6815) ccw projected
  circle A7 centre (48.1191, -214.6815) radius 4.5085
  circle A8 centre (-38.2409, -49.5815) radius 4.5085
  circle A9 centre (-38.2409, -49.5815) radius 1.9939 projected
  circle A10 centre (43.0391, -49.5815) radius 4.5085
  circle A11 centre (43.0391, -49.5815) radius 1.9939 projected
  point P0 (0, 0)
  dimension "d110" = 9.017
  dimension "d111" = 9.017
  dimension "d112" = 9.017
  dimension "d113" = 9.017
  dimension "d120" = 9.017
  dimension "d121" = 0
  dimension "d122" = 0
  dimension "d123" = 9.017
  dimension "d124" = 0
  dimension "d125" = 0
  constraints: 6 centre point, 4 coincident
  measures "d110" diameter of A1
  measures "d111" diameter of A3
  measures "d112" diameter of A5
  measures "d113" diameter of A7
  measures "d120" diameter of A8
  measures "d121" distance of A9.centre A8.centre
  measures "d122" distance of A9.centre A8.centre
  measures "d123" diameter of A10
  measures "d124" distance of A11.centre A10.centre
  measures "d125" distance of A11.centre A10.centre
extrude "Extrusion11" cut sketch "Sketch19" against normal blind 5 contours A1 | A3 | A4 | A5 | A7 | A8 | A9 | A10 | A11
sketch "Sketch20" plane through (0, -205.7831, -50.0038) normal (0, -1, 0) x (1, 0, 0)
  circle A0 centre (18.288, 65.4174) radius 2.032
  line L0 (20.32, 98.425) -> (0, 98.425) projected
  line L1 (20.32, 95.25) -> (20.32, 53.2892) projected
  point P0 (0, 50.0038)
  dimension "d126" = 4.064
  dimension "d127" = 33.0076
  dimension "d128" = 2.032
  constraints: 1 centre point
  measures "d126" diameter of A0
  measures "d127" distance from line of L0 A0.centre
  measures "d128" distance from line of L1 A0.centre
extrude "Extrusion12" cut sketch "Sketch20" against normal blind 13.97